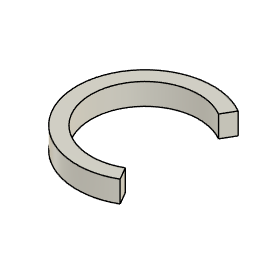
Lock Nat (Autodesk Fusion 360 design; units mm, degrees)
Autodesk Fusion 360 part; units mm, degrees
sketch "スケッチ1" plane through (0, 0, 0) normal (0, 0, 1) x (1, 0, 0)
  circle A0 centre (0, 0) radius 7.5
  circle A1 centre (0, 0) radius 9.5
  line L0 (0, 0) -> (8, 0) construction
  line L1 (0, 0) -> (4.75, -8.2272)
  line L2 (0, 0) -> (8, 0) construction
  line L3 (0, 0) -> (4.75, 8.2272)
  line L4 (0, 0) -> (9, 0) construction
  dimension "d1" = 15
  dimension "d2" = 19
  dimension "d4" = 60
  dimension "d7" = 60
  constraint coincident A0.centre A1.centre
  constraint concentric A0 A1
  constraint horizontal L0
  constraint horizontal L2
  constraint coincident A1 L1.end
  constraint horizontal L4
  constraint coincident A1 L3.end
  measures "d1" diameter of A0
  measures "d2" diameter of A1
  measures "d4" angle of L1 L2
  measures "d7" angle of L3 L4
extrude "押し出し1" add sketch "スケッチ1" along normal blind 3 contours A0 A1 L1 L3 picked at (3.6536, -8.0174)
